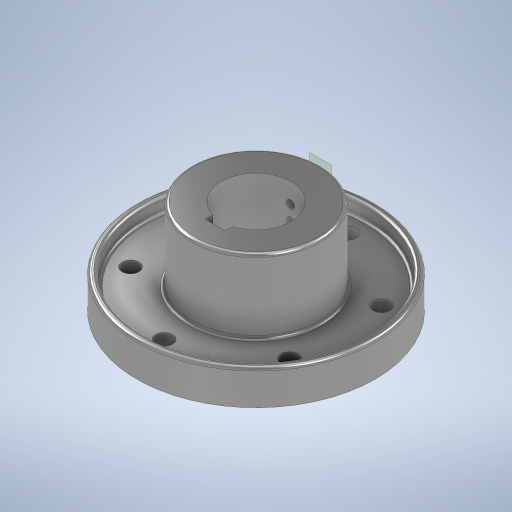
# Autodesk Inventor part: S2spojkav3
Saved by Autodesk Inventor 2023 (Build 270158000, 158)
## iProperties
Created: 2023-05-05
Part Number: S2spojkav3
Material: Sedá litina (42 2420)
Document SubType Name: Modeling
Designer: S21Suk
Density: 7.85 g/cm^3
Appearance: Semi-Polished
Description: Kotoučová spojka
Polotovar: Odlitek
Author: S21Suk
Autodesk Inventor part; units mm, degrees
ref_plane "YZ Plane" through (0, 0, 0) normal (1, 0, 0) x (0, 1, 0)
ref_plane "XZ Plane" through (0, 0, 0) normal (0, 1, 0) x (-1, 0, 0)
ref_plane "XY Plane" through (0, 0, 0) normal (0, 0, 1) x (1, 0, 0)
sketch "Náčrt1" plane through (0, 0, 0) normal (0, 1, 0) x (-1, 0, 0)
  circle A0 centre (0, 0) radius 120
  circle A1 centre (0, 0) radius 112.5
  circle A2 centre (0, 0) radius 35
  circle A3 centre (0, 0) radius 65
  circle A4 centre (0, -92.5) radius 8.5
  line L0 (0, -65) -> (0, -92.5) construction
  circle A5 centre (80.1073, -46.25) radius 8.5
  circle A6 centre (80.1073, 46.25) radius 8.5
  circle A7 centre (0, 92.5) radius 8.5
  circle A8 centre (-80.1073, 46.25) radius 8.5
  circle A9 centre (-80.1073, -46.25) radius 8.5
  dimension "d3" = 130
  dimension "d0" = 240
  dimension "d1" = 225
  dimension "d2" = 70
  dimension "d59" = 17
  dimension "d61" = 27.5
  dimension "d64" = 360
  dimension "d67" = 185
  constraints: 9 centre point, 4 coincident, 2 end point, 1 vertical, 1 vertical alignment, 15 other
  measures "d0" diameter of A0
  measures "d1" diameter of A1
  measures "d2" diameter of A2
  measures "d59" diameter of A4
  measures "d61" distance of L0.start L0.end
  measures "d67" distance of L0.end A7.centre
extrude "Vysunutí1" add sketch "Náčrt1" along normal blind 95 contours A3
extrude "Vysunutí2" add sketch "Náčrt1" along normal blind 21 contours A1
extrude "Vysunutí3" add sketch "Náčrt1" along normal blind 35 contours A0
sketch "Náčrt3" plane through (0, 0, 0) normal (0, -1, 0) x (1, 0, 0)
  line L0 (-10, 41) -> (10, 41)
  line L1 (10, 41) -> (10, 29)
  line L2 (10, 29) -> (-10, 29)
  line L3 (-10, 29) -> (-10, 41)
  circle A0 centre (0, 0) radius 35 projected
  line L4 (-10, 41) -> (10, 29) construction
  line L5 (10, 41) -> (-10, 29) construction
  point P0 (0, 35)
  point P1 (0, 29)
  dimension "d18" = 20
  dimension "d19" = 12
  dimension "d20" = 29
  constraints: 12 end point, 3 midpoint, 2 parallel, 1 horizontal, 1 perpendicular, 1 vertical alignment, 1 other
  measures "d18" distance of L1.end L2.end
  measures "d19" distance between parallel lines of L0 L2
  measures "d20" distance of point (0, 0) point (0, 29)
extrude "Vysunutí5" cut sketch "Náčrt3" against normal through all contours L0 L1 A0 L3 | A0 L1 L2 L3 picked at (1.1251, 30.9456)
fillet "Fillet1" radius 3 5 edges at (112.5, 21, 0) (65, 21, 0) (112.5, 35, 0) (120, 35, 0) (65, 95, 0)
ref_plane "Work Plane1" through (10, 0, -65) normal (0, 0, -1) x (-1, 0, 0)
sketch "Sketch4" plane through (10, 0, -65) normal (0, 0, -1) x (-1, 0, 0)
  line L0 (10, 0) -> (10, 95)
  line L1 (-25, 95) -> (45, 95) projected
  circle A0 centre (10, 60) radius 4
  line L2 (130, 0) -> (-110, 0) projected
  circle A1 centre (10, 75) radius 4
  point P0 (20, 95)
  point P1 (0, 95)
  dimension "d35" = 60
  dimension "d45" = 8
  dimension "d47" = 15
  constraints: 2 centre point, 2 end point, 2 point on line, 1 equal radius, 1 midpoint
  measures "d35" distance from line of L2 A0.centre
  measures "d45" diameter of A0
  measures "d47" distance of A1.centre A0.centre
extrude "Extrusion6" cut sketch "Sketch4" against normal blind 35
thread "Závit3" size "M8x1.25" class "6H" standard "ANSI Metric M Profile" full length
thread "Závit4" size "M8x1.25" class "6H" standard "ANSI Metric M Profile" full length
